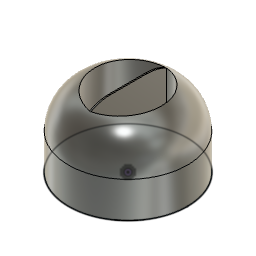
_Roller motor connector.55004d22-41e6-4f78-93e1-cf13529271f8 (Autodesk Fusion 360 design; units mm, degrees)
Autodesk Fusion 360 part; units mm, degrees
note: some values were not read from the file. Set by a fixed rule: which sketch regions a step uses.
sketch "Sketch1" plane through (0, 0, 0) normal (0, 0, 1) x (1, 0, 0)
  circle A0 centre (0, 0) radius 11.625
  dimension "d1" = 23.25
  constraint coincident A0.centre origin
  measures "d1" diameter of A0
extrude "Extrude1" add sketch "Sketch1" along normal blind 15
sketch "Sketch2" plane through (0, 0, 15) normal (0, 0, 1) x (-1, 0, 0)
  circle A0 centre (0, 0) radius 11.625
  circle A1 centre (1, 0) radius 7.5
  circle A2 centre (-1, 0) radius 7.5
  line L0 (-0.125, -9) -> (0.125, -9)
  line L1 (0.125, -9) -> (0.125, 9)
  line L2 (0.125, 9) -> (-0.125, 9)
  line L3 (-0.125, 9) -> (-0.125, -9)
  line L4 (-0.125, -9) -> (0.125, 9) construction
  line L5 (0.125, -9) -> (-0.125, 9) construction
  dimension "d4" = 15
  dimension "d5" = 15
  dimension "d6" = 0.25
  dimension "d7" = 18
  constraint horizontal L0
  constraint perpendicular L0 L1
  constraint parallel L0 L2
  constraint parallel L1 L3
  constraint coincident L4 A0.centre
  constraint coincident L5 A0.centre
  constraint coincident A0.centre origin
  measures "d4" diameter of A1
  measures "d5" diameter of A2
  measures "d6" distance of L1.end L2.end
  measures "d7" distance of L0.end L1.end
extrude "Extrude2" cut sketch "Sketch2" against normal blind 10 contours A2 L1 | A1 L3
fillet "Fillet1" radius 8 1 edges at (-10.8383, -4.2038, 15)
sketch "Sketch4" plane through (0, 0, 0) normal (0, 0, -1) x (1, 0, 0)
  circle A0 centre (0, 0) radius 11.625
  line L0 (-5.75, -5.75) -> (5.75, -5.75)
  line L1 (5.75, -5.75) -> (5.75, 5.75)
  line L2 (5.75, 5.75) -> (-5.75, 5.75)
  line L3 (-5.75, 5.75) -> (-5.75, -5.75)
  line L4 (-5.75, -5.75) -> (5.75, 5.75) construction
  line L5 (5.75, -5.75) -> (-5.75, 5.75) construction
  circle A1 centre (5.75, -5.75) radius 1
  circle A2 centre (-5.75, -5.75) radius 1
  circle A3 centre (5.75, 5.75) radius 1
  circle A4 centre (-5.75, 5.75) radius 1
  dimension "d12" = 11.5
  dimension "d13" = 11.5
  dimension "d14" = 2
  dimension "d15" = 2
  dimension "d16" = 2
  dimension "d17" = 2
  constraint horizontal L0
  constraint perpendicular L0 L1
  constraint parallel L0 L2
  constraint parallel L1 L3
  constraint coincident L4 A0.centre
  constraint coincident L5 A0.centre
  constraint coincident A0.centre origin
  constraint coincident L0.end L1.start
  constraint coincident L0.start L3.end
  constraint coincident L1.end L2.start
  constraint coincident L2.end L3.start
  measures "d12" distance of L1.end L2.end
  measures "d13" distance of L0.end L1.end
  measures "d14" diameter of A1
  measures "d15" diameter of A2
  measures "d16" diameter of A3
  measures "d17" diameter of A4
extrude "Extrude3" cut sketch "Sketch4" against normal blind 3 contours L0 L3 A2 | L0 L3 A2 | L0 L1 A1 | L0 L1 A1 | L2 L3 A4 | L2 L3 A4 | L1 L2 A3 | L1 L2 A3
